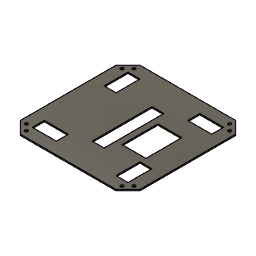
2 bottom base v2 (Autodesk Fusion 360 design; units mm, degrees)
Autodesk Fusion 360 part; units mm, degrees
sketch "Sketch1" plane through (0, 0, 0) normal (0, 0, 1) x (1, 0, 0)
  line L0 (-80, -100) -> (80, -100)
  line L1 (100, -80) -> (100, 80)
  line L2 (80, 100) -> (-80, 100)
  line L3 (-100, 80) -> (-100, -80)
  line L4 (-80, -100) -> (-100, -80)
  line L5 (80, -100) -> (100, -80)
  line L6 (100, 80) -> (80, 100)
  line L7 (-80, 100) -> (-100, 80)
  circle A0 centre (-80, -90) radius 2.5
  circle A1 centre (-90, -80) radius 2.5
  circle A2 centre (80, 90) radius 2.5
  circle A3 centre (90, 80) radius 2.5
  circle A4 centre (-80, 90) radius 2.5
  circle A5 centre (-90, 80) radius 2.5
  circle A6 centre (80, -90) radius 2.5
  circle A7 centre (90, -80) radius 2.5
  line L8 (80, 80) -> (40, 80)
  line L9 (40, 80) -> (40, 60)
  line L10 (40, 60) -> (80, 60)
  line L11 (80, 60) -> (80, 80)
  line L12 (-80, 80) -> (-60, 80)
  line L13 (-60, 80) -> (-60, 40)
  line L14 (-60, 40) -> (-80, 40)
  line L15 (-80, 40) -> (-80, 80)
  line L16 (-10, -50) -> (10, -50)
  line L17 (10, -50) -> (10, 50)
  line L18 (10, 50) -> (-10, 50)
  line L19 (-10, 50) -> (-10, -50)
  line L20 (-80, -80) -> (-40, -80)
  line L21 (-40, -80) -> (-40, -60)
  line L22 (-40, -60) -> (-80, -60)
  line L23 (-80, -60) -> (-80, -80)
  line L24 (80, -80) -> (60, -80)
  line L25 (60, -80) -> (60, -40)
  line L26 (60, -40) -> (80, -40)
  line L27 (80, -40) -> (80, -80)
  line L28 (60, -30) -> (20, -30)
  line L29 (20, -30) -> (20, 30)
  line L30 (20, 30) -> (60, 30)
  line L31 (60, 30) -> (60, -30)
  point P0 (-100, -100)
  point P1 (100, -100)
  point P2 (100, 100)
  point P3 (-100, 100)
  dimension "d1" = 200
  dimension "d2" = 200
  dimension "d3" = 20
  dimension "d4" = 20
  dimension "d5" = 20
  dimension "d6" = 20
  dimension "d7" = 20
  dimension "d8" = 20
  dimension "d9" = 20
  dimension "d10" = 20
  dimension "d11" = 5
  dimension "d12" = 5
  dimension "d13" = 5
  dimension "d14" = 5
  dimension "d15" = 5
  dimension "d16" = 5
  dimension "d17" = 5
  dimension "d18" = 5
  dimension "d19" = 40
  dimension "d20" = 20
  dimension "d21" = 20
  dimension "d22" = 40
  dimension "d27" = 20
  dimension "d28" = 100
  dimension "d29" = 40
  dimension "d30" = 20
  dimension "d31" = 20
  dimension "d32" = 40
  dimension "d33" = 40
  dimension "d34" = 60
  constraint horizontal L0
  constraint vertical L1
  constraint horizontal L2
  constraint vertical L3
  constraint coincident P0 L0
  constraint coincident P0 L3
  constraint coincident P1 L0
  constraint coincident P1 L1
  constraint coincident P2 L1
  constraint coincident P2 L2
  constraint coincident P3 L2
  constraint coincident P3 L3
  constraint horizontal L8
  constraint vertical L9
  constraint horizontal L10
  constraint vertical L11
  constraint horizontal L12
  constraint vertical L13
  constraint horizontal L14
  constraint vertical L15
  constraint horizontal L16
  constraint vertical L17
  constraint horizontal L18
  constraint vertical L19
  constraint horizontal L20
  constraint vertical L21
  constraint horizontal L22
  constraint vertical L23
  constraint horizontal L24
  constraint vertical L25
  constraint horizontal L26
  constraint vertical L27
  constraint horizontal L28
  constraint vertical L29
  constraint horizontal L30
  constraint vertical L31
  measures "d1" distance of P0 P1
  measures "d2" distance of P0 P3
  measures "d3" distance of P0 L0.start
  measures "d4" distance of P0 L3.end
  measures "d5" distance of P1 L0.end
  measures "d6" distance of P1 L1.start
  measures "d7" distance of P2 L1.end
  measures "d8" distance of P2 L2.start
  measures "d9" distance of P3 L2.end
  measures "d10" distance of P3 L3.start
  measures "d11" diameter of A0
  measures "d12" diameter of A1
  measures "d13" diameter of A2
  measures "d14" diameter of A3
  measures "d15" diameter of A4
  measures "d16" diameter of A5
  measures "d17" diameter of A6
  measures "d18" diameter of A7
  measures "d19" distance of L8.start L8.end
  measures "d20" distance of L8.start L10.end
  measures "d21" distance of L12.start L12.end
  measures "d22" distance of L12.start L14.end
  measures "d27" distance of L16.start L16.end
  measures "d28" distance of L16.start L18.end
  measures "d29" distance of L20.start L20.end
  measures "d30" distance of L20.start L22.end
  measures "d31" distance of L24.start L24.end
  measures "d32" distance of L24.start L26.end
  measures "d33" distance of L28.start L28.end
  measures "d34" distance of L28.start L30.end
extrude "Extrude1" add sketch "Sketch1" along normal blind 2
equation "d4 = d3"
equation "d6 = d5"
equation "d8 = d7"
equation "d10 = d9"
